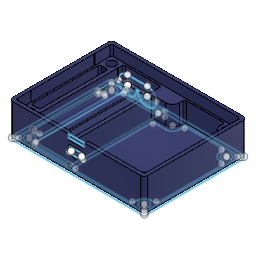
iot-data-logger-enclosure-bottom-base v35 (Autodesk Fusion 360 design; units mm, degrees)
Autodesk Fusion 360 part; units mm, degrees
sketch "Sketch1" plane through (0, 0, 0) normal (0, 1, 0) x (1, 0, 0)
  line L0 (2, 0) -> (77, 0)
  line L1 (0, -58) -> (0, -2)
  arc A0 (79, -1.0015) -> (79, -0.9985) centre (78, -1) ccw
  arc A1 (79, -59.0008) -> (79, -58.9992) centre (78, -59) ccw
  arc A2 (0.9987, -60) -> (1.0013, -60) centre (1, -59) ccw
  circle A3 centre (6, -6) radius 2.5
  line L2 (3, -2) -> (76, -2)
  line L3 (77, -2.9998) -> (77, -57.0015)
  line L4 (76, -58) -> (3, -58)
  line L5 (2, -57) -> (2, -3)
  arc A4 (3, -2) -> (2, -3) centre (3, -3) ccw
  line L6 (3, -2) -> (10, -2)
  line L7 (10, -4) -> (10, -6)
  line L8 (6, -10) -> (4, -10)
  line L9 (2, -10) -> (2, -3)
  arc A5 (2, -11.6976) -> (2, -12.3562) centre (4, -12.0269) ccw
  circle A6 centre (6, -54) radius 2.5
  line L10 (4, -50) -> (6, -50)
  line L11 (10, -54) -> (10, -56)
  arc A7 (2, -48.9994) -> (2, -49.0006) centre (3, -49) ccw
  arc A8 (11, -58) -> (11.0013, -58) centre (11, -57) ccw
  line L12 (69, -56) -> (69, -54)
  line L13 (75, -50) -> (73, -50)
  line L14 (3, -49) -> (3, -10.9995)
  arc A9 (11, -3) -> (10, -4) centre (11, -4) ccw
  arc A10 (4, -10) -> (3, -10.9995) centre (4, -11) ccw
  arc A11 (3, -49) -> (4, -50) centre (4, -49) ccw
  arc A12 (10, -56) -> (11.0013, -57) centre (11, -56) ccw
  arc A13 (2, -57) -> (3, -58) centre (3, -57) ccw
  circle A14 centre (73, -54) radius 2.5
  arc A15 (75, -50) -> (76, -49) centre (75, -49) ccw
  arc A16 (68, -57) -> (69, -56) centre (68, -56) ccw
  arc A17 (73, -50) -> (69, -54) centre (73, -54) ccw
  arc A18 (76, -58) -> (77, -56.9985) centre (76, -57) ccw
  line L15 (69, -6) -> (69, -4)
  line L16 (73, -10) -> (75, -10)
  circle A19 centre (73, -6) radius 2.5
  arc A20 (69, -4) -> (68, -3) centre (68, -4) ccw
  arc A21 (76, -11) -> (75, -10) centre (75, -11) ccw
  line L17 (76, -11) -> (76, -49)
  arc A22 (69, -6) -> (73, -10) centre (73, -6) ccw
  arc A23 (77, -6.003) -> (77, -5.997) centre (73, -6) ccw
  arc A24 (77, -2.9998) -> (76, -2) centre (76, -3) ccw
  line L18 (11, -3) -> (31, -3)
  line L19 (32, -3.9993) -> (32, -56)
  line L20 (10, -56) -> (10, -4)
  arc A25 (32, -4.0007) -> (32, -3.9993) centre (31, -4) ccw
  line L21 (10, -4) -> (10, -4)
  line L22 (10, -4) -> (10, -6)
  line L23 (10, -6) -> (10, -6)
  line L24 (10, -6) -> (10, -4)
  line L25 (32, -4.0007) -> (10, -4.0007)
  line L26 (10, -4.0007) -> (10, -5.5007)
  line L27 (10, -5.5007) -> (32, -5.5007)
  line L28 (32, -5.5007) -> (32, -4.0007)
  line L29 (10, -56) -> (32, -56)
  line L30 (32, -56) -> (32, -54.5)
  line L31 (32, -54.5) -> (10, -54.5)
  line L32 (10, -54.5) -> (10, -56)
  line L33 (11.0013, -57) -> (10.9987, -57)
  arc A26 (31, -57) -> (32, -56) centre (31, -56) ccw
  line L34 (11, -3) -> (31, -3)
  line L35 (46.5, -3) -> (68, -3)
  arc A27 (32, -4.0007) -> (31, -3) centre (31, -4) ccw
  arc A28 (34, -3.9998) -> (34, -4.0002) centre (35, -4) ccw
  arc A29 (34, -55.9992) -> (35, -57) centre (35, -56) ccw
  line L36 (68, -57) -> (35, -57)
  line L37 (31, -57) -> (10.9998, -57)
  line L38 (10, -6.5) -> (9.9686, -6.5)
  line L39 (8, -11) -> (8, -49)
  line L40 (10, -54.5) -> (10, -6.5)
  line L41 (6, -50) -> (7, -50)
  arc A30 (7, -50) -> (8, -49) centre (7, -49) ccw
  line L42 (5.5, -10) -> (7, -10)
  arc A31 (9.9686, -6.5) -> (10, -6) centre (6, -6) ccw
  arc A32 (8, -11) -> (7, -10) centre (7, -11) ccw
  line L43 (37.5, -10) -> (35, -10)
  line L44 (45.5, -6) -> (45.5, -4)
  line L45 (34, -3.9998) -> (34, -4.0002)
  line L46 (34, -10.9998) -> (34, -56.0008)
  line L47 (37.5, -10) -> (41.5, -10)
  arc A33 (41.5, -10) -> (45.5, -6) centre (41.5, -6) ccw
  arc A34 (35, -10) -> (34, -11.0002) centre (35, -11) ccw
  arc A35 (46.5, -3) -> (45.5, -4) centre (46.5, -4) ccw
  arc A36 (2, 0) -> (0, -2) centre (2, -2) ccw
  arc A37 (0, -58) -> (2, -60) centre (2, -58) ccw
  line L48 (77, -60) -> (2, -60)
  line L49 (1.0013, -60) -> (0.9987, -60)
  arc A38 (77, -60) -> (79, -57.9989) centre (77, -58) ccw
  line L50 (79, -58.9992) -> (79, -59.0008)
  line L51 (79, -0.9985) -> (79, -1.0015)
  line L52 (79, -1.9978) -> (79, -58.0011)
  arc A39 (79, -2.0022) -> (77, 0) centre (77, -2) ccw
  dimension "d9" = 73
  dimension "d13" = 1.5
  dimension "d14" = 1.5
  dimension "d51" = 5
  dimension "d52" = 5
  dimension "d53" = 5
  dimension "d54" = 5
  constraint horizontal L0
  constraint vertical L51
  constraint horizontal L48
  constraint vertical L1
  constraint tangent A1 L48
  constraint tangent L0 A0
  constraint coincident A1.end L51
  constraint coincident A2.end L48
  constraint horizontal L2
  constraint vertical L3
  constraint horizontal L4
  constraint vertical L5
  constraint tangent L2 A4
  constraint horizontal L6
  constraint vertical L7
  constraint horizontal L8
  constraint vertical L9
  constraint coincident L5 A5.end
  constraint coincident L5 A5.start
  constraint perpendicular L4 L11
  constraint tangent L10 A7
  constraint tangent L11 A8
  constraint coincident L5 A7.start
  constraint coincident L4 A8.end
  constraint tangent L2 A22
  constraint horizontal L34
  constraint vertical L14
  constraint tangent L10 A11
  constraint coincident A8.centre A12
  constraint coincident L5 A7.end
  constraint coincident L4 A8.start
  constraint coincident A12 L37.end
  constraint tangent L4 A13
  constraint tangent L4 A18
  constraint coincident L3 A18.end
  constraint coincident A18 L3.end
  constraint tangent L15 A22
  constraint perpendicular L15 L34
  constraint tangent L16 A22
  constraint tangent A20 L34
  constraint tangent L2 A24
  constraint concentric A19 A22
  constraint coincident L3 A23.start
  constraint concentric A22 A23
  constraint coincident L3 A23.end
  constraint horizontal L18
  constraint vertical L19
  constraint vertical L20
  constraint perpendicular L36 L45
  constraint tangent L18 A25
  constraint tangent A25 L34
  constraint coincident L19 A25.start
  constraint vertical L22
  constraint vertical L24
  constraint horizontal L25
  constraint vertical L26
  constraint horizontal L27
  constraint vertical L28
  constraint horizontal L29
  constraint vertical L30
  constraint horizontal L31
  constraint vertical L32
  constraint coincident L29 A26.centre
  constraint coincident A12 L33.end
  constraint concentric A25 A27
  constraint tangent L18 A27
  constraint collinear L34 L35
  constraint tangent L35 A28
  constraint tangent A29 L36
  constraint coincident A29.start L45
  constraint collinear L36 L37
  constraint coincident A29 L46.end
  constraint horizontal L38
  constraint vertical L39
  constraint vertical L40
  constraint coincident L20 L38.start
  constraint tangent L39 A30
  constraint tangent L42 A32
  constraint perpendicular L43 L44
  constraint tangent L43 A34
  constraint collinear L45 L46
  constraint perpendicular L2 L44
  constraint tangent L47 A33
  constraint coincident L46 A34.end
  constraint coincident A34 L46.start
  constraint tangent L0 A36
  constraint tangent A37 L48
  constraint collinear L48 L49
  constraint tangent L48 A38
  constraint coincident A38.end L51
  constraint coincident A38 L52.end
  constraint collinear L50 L51
  constraint tangent L0 A39
  constraint coincident L52.start A39
  constraint collinear L51 L52
  constraint coincident L52 A39.start
  measures "d9" distance of A4.centre A24.centre
  measures "d13" distance of A25.start L27.end
  measures "d14" distance of L11.end L31.end
  measures "d51" diameter of A14
  measures "d52" diameter of A6
  measures "d53" diameter of A3
  measures "d54" diameter of A19
sketch "Sketch2" plane through (0, 0, 0) normal (0, 0, 1) x (1, 0, 0)
  line L0 (10, 0, 1) -> (32, 0, 1)
  arc A0 through (21.5, 7.25, 6) (26.75, 2, 6) (32, 7.25, 6)
  arc A1 through (10, 7.25, 6) (15.25, 2, 6) (20.5, 7.25, 6)
  line L1 (20.5, 7.25, 6) -> (21.5, 7.25, 6)
  line L2 (26.75, 7.25, 6) -> (26.75, 7.25, 6)
  line L3 (21.5, 7.25, 6) -> (20.5, 7.25, 6)
  line L4 (15.25, 7.25, 6) -> (15.25, 7.25, 6)
  line L5 (20.5, 7.25, 6) -> (21.5, 7.25, 6)
  line L6 (26.75, 12.4998, 6) -> (15.25, 12.4998, 6)
  arc A2 through (21.5, 7.25, 6) (30.4775, 3.5529, 6) (26.707, 12.4998, 6)
  arc A3 through (15.293, 12.4998, 6) (11.5225, 3.5529, 6) (20.5, 7.25, 6)
extrude "Extrude1" add sketch "Sketch1" along normal blind 2 contours L12 L13 A15 A16 A17 L15 L16 A20 A21 L17 A22 L35 A29 L36 L43 L44 L46 L47 A33 A34 A35 makes body 1
extrude "Extrude2" add sketch "Sketch1" along normal blind 2 separate body contours L8 L10 A7 L14 A10 A11 L39 L41 A30 L42 A32 | A7 L14 A11 picked at (3.3371, -49.0497) makes body 2
extrude "Extrude3" add sketch "Sketch1" along normal blind 19.5 separate body contours L0 L1 A1 A36 A37 L48 A38 L52 A39 | A1 A38 picked at (78.0382, -59.0382) makes body 3
extrude "Extrude4" add sketch "Sketch1" along normal blind 13.5 contours A7 L14 A11 | A8 A12 L33 L37 | L2 L3 L4 L5 A4 L6 L9 A13 A18 A23 A24 | A28 picked at (2.3519, -49.1479) picked at (10.9499, -57.6629) bodies 1 2 3
extrude "Extrude5" add sketch "Sketch1" along normal blind 2 contours A8 A12 L29 | A8 A12 L33 L37 | A8 L29 A26 L37 | A25 L25 A27 | A9 L18 A25 L25 L34 picked at (10.9499, -56.3371) bodies 1
extrude "Extrude6" add sketch "Sketch1" along normal blind 7.25 contours L7 L19 L20 L22 L24 L25 L26 L27 L28 | L7 L11 L19 L20 L22 L24 L27 L31 L40 | L11 L19 L20 L29 L30 L31 L32 bodies 1
fillet "Fillet1" radius 1 8 edges at (78.415, 0, 0.5866) (39.5, 0, 0) (0.5858, 0, 0.5858) (0, 0, 30) (0.5858, 0, 59.4142) (39.5, 0, 60) (78.4138, 0, 59.4146) (79, 0, 30.0016) on bodies 1
extrude "Extrude13" cut sketch "Sketch2" along normal blind 48 contours A0 A1 L1 L3 L5 L6 A2 A3 in plane through (0, 0, 6) normal (0, 0, 1) bodies 1
extrude "Extrude14" add sketch "Sketch1" along normal blind 8 separate body contours A3 | A6 | A14 | A19 makes body 4 at (75.4969, 5.3333, 54.1246) makes body 5 at (75.4969, 5.3333, 6.1246) makes body 6 at (8.4969, 5.3333, 54.1246) makes body 7 at (8.4969, 5.3333, 6.1246)
combine "Combine4" operation add target body 1 tool bodies 4 6 7 5
sketch "Sketch3" plane through (0, 0, 0) normal (0, 0, 1) x (1, 0, 0)
  line L0 (36.5, 10, 60) -> (42.5, 10, 60)
  line L1 (44, 11.5, 60) -> (44, 12, 60)
  line L2 (42.5, 13.5, 60) -> (36.5, 13.5, 60)
  line L3 (35, 12, 60) -> (35, 11.5, 60)
  arc A0 through (44, 12, 60) (43.5607, 13.0607, 60) (42.5, 13.5, 60)
  arc A1 through (42.5, 10, 60) (43.5607, 10.4393, 60) (44, 11.5, 60)
  arc A2 through (36.5, 13.5, 60) (35.4393, 13.0607, 60) (35, 12, 60)
  arc A3 through (35, 11.5, 60) (35.4393, 10.4393, 60) (36.5, 10, 60)
  line L4 (35, 19.5, 60) -> (44, 19.5, 60)
  line L5 (44, 19.5, 60) -> (44, 17.5, 60)
  line L6 (44, 17.5, 60) -> (35, 17.5, 60)
  line L7 (35, 17.5, 60) -> (35, 19.5, 60)
  point P0 (35.5, 10.75)
  point P1 (43.5, 10.75)
  dimension "d66" = 9
  dimension "d67" = 2
extrude "Extrude15" cut sketch "Sketch3" against normal blind 3 contours L0 L1 L2 L3 A0 A1 A2 A3 in plane through (0, 0, 60) normal (0, 0, 1) bodies 1
fillet "Fillet2" radius 0.5 7 edges at (35.4393, 13.0607, 57) (35, 11.75, 57) (35.4393, 10.4393, 57) (39.5, 10, 57) (43.5607, 10.4393, 57) (44, 11.75, 57) (43.5607, 13.0607, 57) on bodies 1
fillet "Fillet3" radius 1 8 edges at (44, 11.75, 60) (43.5607, 10.4393, 60) (39.5, 10, 60) (35.4393, 10.4393, 60) (35, 11.75, 60) (35.4393, 13.0607, 60) (39.5, 13.5, 60) (43.5607, 13.0607, 60) on bodies 1
extrude "Extrude16" cut sketch "Sketch3" against normal blind 2 contours L4 L5 L6 L7 in plane through (0, 0, 60) normal (0, 0, 1) bodies 1
fillet "Fillet4" radius 1 1 edges at (39.5, 17.5, 60) on bodies 1
fillet "Fillet5" radius 1 1 edges at (35, 18.5, 58) on bodies 1
fillet "Fillet6" radius 1 1 edges at (44, 18.5, 58) on bodies 1
named bodies: "bottom-cover"
